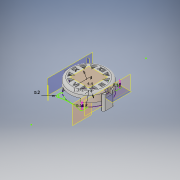
# Autodesk Inventor part: watchBodyOneTopV1.1
Saved by Autodesk Inventor 2019 (Build 230136000, 136)
## iProperties
Created: 2019-10-08
Part Number: watchBodyOneTopV1.1
Material: Generic
Document SubType Name: Modeling
Designer: Derek
Density: 1 g/cm^3
Appearance: Default
Author: Derek
Autodesk Inventor part; units mm, degrees
ref_plane "YZ Plane" through (0, 0, 0) normal (1, 0, 0) x (0, 1, 0)
ref_plane "XZ Plane" through (0, 0, 0) normal (0, 1, 0) x (-1, 0, 0)
ref_plane "XY Plane" through (0, 0, 0) normal (0, 0, 1) x (1, 0, 0)
sketch "Sketch1" plane through (0, 0, 0) normal (0, 1, 0) x (-1, 0, 0)
  circle A0 centre (0, 0) radius 22
  arc A1 (-13.7238, -17.1947) -> (13.7238, -17.1947) centre (0, 0) ccw
  dimension "d0" = 44
  dimension "d11" = 13.7238
  constraints: 4 point on circle, 2 centre point, 1 coincident, 1 concentric
  measures "d0" diameter of A0
  measures "d11" horizontal distance of point (0, 0) A0.start
ref_plane "Work Plane10" through (0, 7, 0) normal (0, 1, 0) x (1, 0, 0)
sketch "Sketch5" plane through (0, 7, 0) normal (0, 1, 0) x (1, 0, 0)
  circle A0 centre (0, 0) radius 20
  dimension "d8" = 40
  constraints: 1 centre point, 1 coincident
  measures "d8" diameter of A0
ref_plane "Work Plane9" through (0, 0, 0) normal (0, -1, 0) x (1, 0, 0)
sketch "Sketch8" plane through (0, 0, 0) normal (0, -1, 0) x (1, 0, 0)
  arc A0 (-11.5874, -18.7011) -> (11.5874, -18.7011) centre (0, 0) ccw
  line L0 (-15.0453, -16.0511) -> (-15.0453, -22.0257)
  line L1 (15.0453, -16.0511) -> (15.0453, -22.0257)
  arc A1 (-15.0453, -16.0511) -> (15.0453, -16.0511) centre (0, 0) ccw
  arc A2 (-15.0453, -22.0257) -> (-13.0453, -24.0257) centre (-13.0453, -22.0257) ccw
  arc A3 (13.0453, -24.0257) -> (15.0453, -22.0257) centre (13.0453, -22.0257) ccw
  line L2 (-15.0451, -16.0514) -> (-15.0451, -22.026)
  arc A4 (-15.0451, -22.026) -> (-13.0451, -24.026) centre (-13.0451, -22.026) ccw
  arc A5 (13.0456, -24.026) -> (15.0456, -22.026) centre (13.0456, -22.026) ccw
  line L3 (15.0456, -16.0514) -> (15.0456, -22.026)
  arc A6 (-15.0451, -16.0514) -> (15.0456, -16.0514) centre (0.0003, -0.0002) ccw
  arc A7 (13.0456, -24.026) -> (-13.0451, -24.026) centre (0.0003, -66.8475) ccw
  point P0 (0, 0)
  point P1 (0, 0)
  constraints: 16 point on circle, 8 centre point, 8 end point
ref_plane "Work Plane8" through (0, 0, 0) normal (0, -1, 0) x (1, 0, 0)
sketch "Sketch11" plane through (0, 0, 0) normal (0, -1, 0) x (1, 0, 0)
  arc A0 (11.5874, 18.7011) -> (-11.5874, 18.7011) centre (0, 0) ccw
  line L0 (-15.0453, 16.0511) -> (-15.0453, 22.0257)
  line L1 (15.0453, 16.0511) -> (15.0453, 22.0257)
  arc A1 (15.0453, 16.0511) -> (-15.0453, 16.0511) centre (0, 0) ccw
  arc A2 (-13.0453, 24.0257) -> (-15.0453, 22.0257) centre (-13.0453, 22.0257) ccw
  arc A3 (15.0453, 22.0257) -> (13.0453, 24.0257) centre (13.0453, 22.0257) ccw
  line L2 (-15.0451, 16.0514) -> (-15.0451, 22.026)
  arc A4 (-13.0451, 24.026) -> (-15.0451, 22.026) centre (-13.0451, 22.026) ccw
  arc A5 (15.0456, 22.026) -> (13.0456, 24.026) centre (13.0456, 22.026) ccw
  line L3 (15.0456, 16.0514) -> (15.0456, 22.026)
  arc A6 (15.0456, 16.0514) -> (-15.0451, 16.0514) centre (0.0003, 0.0002) ccw
  arc A7 (-13.0451, 24.026) -> (13.0456, 24.026) centre (0.0003, 66.8475) ccw
  point P0 (0, 0)
  dimension "d27" = 2
  dimension "d28" = 2
  constraints: 16 point on circle, 8 centre point, 8 end point, 4 tangent, 4 vertical, 2 equal radius
  measures "d27" radius of A2
  measures "d28" radius of A4
ref_plane "Work Plane5" through (14.0456, 0, 22.026) normal (1, 0, 0) x (0, 0, -1)
sketch "Sketch14" plane through (14.0456, 0, 22.026) normal (1, 0, 0) x (0, 0, -1)
  line L0 (0, 0) -> (0, 7) projected
  circle A0 centre (0, 3.5) radius 0.9
  point P0 (22.026, 0)
  dimension "d38" = 1.8
  constraints: 1 centre point, 1 midpoint
  measures "d38" diameter of A0
ref_plane "Work Plane6" through (14.0456, 0, 22.026) normal (1, 0, 0) x (0, 0, -1)
sketch "Sketch15" plane through (14.0456, 0, 22.026) normal (1, 0, 0) x (0, 0, -1)
  line L0 (44.1089, 7) -> (44.1089, 0) projected
  circle A0 centre (44.1089, 3.5) radius 0.9
  point P0 (22.026, 0)
  dimension "d41" = 1.8
  constraints: 1 centre point, 1 midpoint
  measures "d41" diameter of A0
ref_plane "Work Plane7" through (0, 7, 0) normal (0, 1, 0) x (1, 0, 0)
sketch "Sketch16" plane through (0, 7, 0) normal (0, 1, 0) x (1, 0, 0)
  circle A0 centre (0, 0) radius 22
  circle A1 centre (0, -0.3745) radius 18.85
  dimension "d44" = 37.7
  constraints: 2 centre point, 1 coincident
  measures "d44" diameter of A1
extrude "Extrusion13" add sketch "Sketch16" along normal blind 7.5
ref_plane "Work Plane3" through (22, 0, 0) normal (1, 0, 0) x (0, 1, 0)
sketch "Sketch17" plane through (22, 0, 0) normal (1, 0, 0) x (0, 1, 0)
  line L0 (7, -18.2255) -> (7, 18.9745) projected
  line L1 (11.1125, 6.35) -> (7, 6.35)
  line L2 (7, 6.35) -> (7, -6.5465)
  line L3 (7, -6.5465) -> (11.1125, -6.5465)
  line L4 (11.1125, -6.5465) -> (11.1125, 6.35)
  constraints: 8 end point, 2 parallel, 1 horizontal, 1 perpendicular, 1 point on line
extrude "Extrusion14" add sketch "Sketch17" along normal mid plane 3
ref_plane "Work Plane12" through (21.0034, 7, -6.5465) normal (0, -1, 0) x (1, 0, 0)
sketch "Sketch18" plane through (21.0034, 7, -6.5465) normal (0, -1, 0) x (1, 0, 0)
  arc A0 (-35.8073, -9.7276) -> (-35.8073, 22.8206) centre (-21.0034, 6.5465) ccw projected
  line L0 (0, 0) -> (2.4966, 0) projected
  line L1 (0, 0) -> (2.4966, 0)
  line L2 (2.4966, 12.8965) -> (0.0602, 12.8965) projected
  line L3 (2.4966, 0) -> (2.4966, 12.8965)
  line L4 (2.4966, 12.8965) -> (0.0602, 12.8965)
  arc A1 (0, 0) -> (0.0602, 12.8965) centre (-21.0034, 6.5465) ccw
  constraints: 6 end point, 3 point on circle, 2 collinear, 1 centre point, 1 perpendicular
extrude "Extrusion15" add sketch "Sketch18" along normal blind 12.8
ref_plane "Work Plane4" through (-22, 0, 0) normal (-1, 0, 0) x (0, -1, 0)
sketch "Sketch19" plane through (-22, 0, 0) normal (-1, 0, 0) x (0, -1, 0)
  line L0 (-11.1125, -6.5465) -> (-11.1125, 6.35) projected
  line L1 (-7, -20) -> (-7, 20) projected
  line L2 (-11.1125, -6.5465) -> (-7, -6.5465)
  line L3 (-7, -6.5465) -> (-7, 6.35)
  line L4 (-7, 6.35) -> (-11.1125, 6.35)
  line L5 (-11.1125, 6.35) -> (-11.1125, -6.5465)
  point P0 (0, 0)
  constraints: 8 end point, 2 parallel, 1 horizontal, 1 perpendicular, 1 point on line
extrude "Extrusion16" add sketch "Sketch19" along normal mid plane 3
sketch "Sketch20" plane through (-23.5, 7, -6.5465) normal (0, -1, 0) x (1, 0, 0)
  line L0 (0, 0) -> (2.4966, 0) projected
  line L1 (2.4966, 0) -> (0, 0)
  line L2 (0, 12.8965) -> (0, 0) projected
  line L3 (0, 0) -> (0, 12.8965)
  arc A0 (2.4363, 12.8965) -> (2.4966, 0) centre (23.5, 6.5465) ccw projected
  line L4 (0, 12.8965) -> (2.4363, 12.8965)
  point P0 (3, 0)
  constraints: 6 end point, 2 collinear, 1 perpendicular
extrude "Extrusion17" add sketch "Sketch20" along normal blind 12.8
ref_plane "Work Plane11" through (0, 14.5, 0) normal (0, 1, 0) x (1, 0, 0)
sketch "Sketch23" plane through (0, 14.5, 0) normal (0, 1, 0) x (1, 0, 0)
  circle A0 centre (0, 0) radius 20
  constraints: 1 centre point, 1 coincident
extrude "Extrusion20" add sketch "Sketch23" against normal blind 2
fillet "Fillet1" radius 3 1 edges at (-22, 14.5, 0)
ref_plane "Work Plane13" through (-21.0034, 11.1125, -21.5465) normal (0, 0, -1) x (-1, 0, 0)
sketch "Sketch36" plane through (23.5, 0, 0) normal (1, 0, 0) x (0, 0, -1)
  line L0 (3.8069, 13.5118) -> (-2.6931, 13.5118)
  line L1 (-2.6931, 13.5118) -> (-2.6931, 7.0118)
  line L2 (-2.6931, 7.0118) -> (3.8069, 7.0118)
  line L3 (3.8069, 7.0118) -> (3.8069, 13.5118)
  point P0 (0, 0)
  dimension "d96" = 6.5
  dimension "d97" = 6.5
  constraints: 8 end point, 2 parallel, 1 horizontal, 1 perpendicular
  measures "d96" distance of L2.end L1.end
  measures "d97" distance of L1.end L0.end
extrude "Extrusion26" cut sketch "Sketch36" against normal blind 5
sketch "Sketch37" plane through (18.5, 0, 0) normal (1, 0, 0) x (0, 0, -1)
  line L0 (3.8069, 13.5118) -> (3.8069, 7.0118) projected
  line L1 (3.8069, 13.5118) -> (-2.6931, 13.5118) projected
  line L2 (3.8069, 7.0118) -> (-2.6931, 7.0118)
  line L3 (-2.6931, 7.0118) -> (-2.6931, 13.5118)
  line L4 (-2.6931, 13.5118) -> (3.8069, 13.5118)
  line L5 (3.8069, 13.5118) -> (3.8069, 7.0118)
  point P0 (0, 0)
  constraints: 8 end point, 2 parallel, 1 horizontal, 1 perpendicular
extrude "Extrusion27" cut sketch "Sketch37" against normal blind 5
fillet "Fillet2" radius 2 1 edges at (-23.5, 2.6562, -6.5465)
fillet "Fillet3" radius 2 1 edges at (-23.5, 2.6562, 6.35)
fillet "Fillet4" radius 2 2 edges at (23.5, 2.6562, 6.35) (23.5, 2.6562, -6.5465)
ref_plane "Work Plane14" through (-21.0637, -5.8, 26.35) normal (0, 0, 1) x (1, 0, 0)
sketch "Sketch39" plane through (0, 7, 0) normal (0, -1, 0) x (1, 0, 0)
  circle A0 centre (0, 0) radius 20
  circle A1 centre (0, 0) radius 19 projected
  circle A2 centre (0, 0) radius 22
  constraints: 2 centre point, 2 coincident
extrude "Extrusion30" add sketch "Sketch39" along normal blind 3 contours A2
sketch "Sketch40" plane through (-21.0637, -5.8, 26.35) normal (0, 0, 1) x (1, 0, 0)
  line L0 (0.0602, 9.8) -> (42.0671, 9.8) projected
  line L1 (31.2191, 9.8) -> (10.2191, 9.8)
  line L2 (10.2191, 9.8) -> (10.2191, 13.8)
  line L3 (10.2191, 13.8) -> (31.2191, 13.8)
  line L4 (31.2191, 13.8) -> (31.2191, 9.8)
  point P0 (21.0637, 5.8)
  dimension "d115" = 21
  dimension "d116" = 4
  constraints: 8 end point, 2 parallel, 1 horizontal, 1 perpendicular, 1 point on line
  measures "d115" distance of L2.end L3.end
  measures "d116" distance of L1.end L2.end
extrude "Extrusion31" cut sketch "Sketch40" against normal blind 12
sketch "Sketch24" plane through (0, 14.5, 0) normal (0, 1, 0) x (1, 0, 0)
  line L0 (10.9767, 13.2796) -> (5.8224, 10.3341)
  line L1 (5.8224, 10.3341) -> (5.8486, 16.2706)
  line L2 (5.8486, 16.2706) -> (10.9767, 13.2796)
  line L3 (16.5131, 5.8755) -> (10.4909, 5.9199)
  line L4 (10.4909, 5.9199) -> (13.5405, 11.113)
  line L5 (13.5405, 11.113) -> (16.5131, 5.8755)
  line L6 (16.5966, -6.2702) -> (13.432, -11.5016)
  line L7 (13.432, -11.5016) -> (10.4838, -6.1453)
  line L8 (10.4838, -6.1453) -> (16.5966, -6.2702)
  line L9 (11.4269, -13.3864) -> (6.4692, -16.6726)
  line L10 (6.4692, -16.6726) -> (6.1021, -10.736)
  line L11 (6.1021, -10.736) -> (11.4269, -13.3864)
  line L12 (-6.0129, -10.6804) -> (-5.9694, -16.6431)
  line L13 (-5.9694, -16.6431) -> (-11.155, -13.6995)
  line L14 (-11.155, -13.6995) -> (-6.0129, -10.6804)
  line L15 (-10.2253, -6.1862) -> (-13.3868, -11.6656)
  line L16 (-13.3868, -11.6656) -> (-16.5514, -6.188)
  line L17 (-16.5514, -6.188) -> (-10.2253, -6.1862)
  line L18 (-10.6525, 5.6862) -> (-16.9579, 5.7959)
  line L19 (-16.9579, 5.7959) -> (-13.7102, 11.2018)
  line L20 (-13.7102, 11.2018) -> (-10.6525, 5.6862)
  line L21 (-6.1885, 9.9631) -> (-11.4992, 13.2741)
  line L22 (-11.4992, 13.2741) -> (-5.9764, 16.2178)
  line L23 (-5.9764, 16.2178) -> (-6.1885, 9.9631)
  line L24 (-3.7539, 17.3089) -> (3.62, 17.3089) construction
  line L25 (3.62, 17.3089) -> (3.62, 12.7336) construction
  line L26 (3.62, 12.7336) -> (-3.7539, 12.7336) construction
  line L27 (-3.7539, 12.7336) -> (-3.7539, 17.3089) construction
  line L28 (5.558, 19.0366) -> (5.558, 14.4613) construction
  line L29 (12.8351, 2.0932) -> (17.8398, 2.0932) construction
  line L30 (17.8398, 2.0932) -> (17.8398, -2.2068) construction
  line L31 (17.8398, -2.2068) -> (12.8351, -2.2068) construction
  line L32 (12.8351, -2.2068) -> (12.8351, 2.0932) construction
  line L33 (-2.7032, -13.1458) -> (2.3586, -13.1458) construction
  line L34 (2.3586, -13.1458) -> (2.3586, -17.8139) construction
  line L35 (2.3586, -17.8139) -> (-2.7032, -17.8139) construction
  line L36 (-2.7032, -17.8139) -> (-2.7032, -13.1458) construction
  line L37 (-18.4501, 2.0895) -> (-13.3883, 2.0895) construction
  line L38 (-13.3883, 2.0895) -> (-13.3883, -2.5786) construction
  line L39 (-13.3883, -2.5786) -> (-18.4501, -2.5786) construction
  line L40 (-18.4501, -2.5786) -> (-18.4501, 2.0895) construction
  line L41 (-18.0404, -2.2105) -> (-18.0404, 2.0895)
  line L42 (-18.0404, 2.0895) -> (-17.1719, 2.0895)
  line L43 (-17.1719, 2.0895) -> (-17.1719, -2.2105)
  line L44 (-17.1719, -2.2105) -> (-18.0404, -2.2105)
  line L45 (-16.7786, -2.2105) -> (-15.294, 0.0279)
  line L46 (-15.294, 0.0279) -> (-16.641, 2.0895)
  line L47 (-16.641, 2.0895) -> (-15.6283, 2.0895)
  line L48 (-15.6283, 2.0895) -> (-14.7761, 0.8047)
  line L49 (-14.7761, 0.8047) -> (-13.924, 2.0895)
  line L50 (-13.924, 2.0895) -> (-12.9113, 2.0895)
  line L51 (-12.9113, 2.0895) -> (-14.2648, 0.0312)
  line L52 (-14.2648, 0.0312) -> (-12.7802, -2.2105)
  line L53 (-12.7802, -2.2105) -> (-13.8289, -2.2105)
  line L54 (-13.8289, -2.2105) -> (-14.7827, -0.7554)
  line L55 (-14.7827, -0.7554) -> (-15.7364, -2.2105)
  line L56 (-15.7364, -2.2105) -> (-16.7786, -2.2105)
  line L57 (-3.736, 13.0089) -> (-2.2514, 15.2474)
  line L58 (-2.2514, 15.2474) -> (-3.5984, 17.3089)
  line L59 (-3.5984, 17.3089) -> (-2.5857, 17.3089)
  line L60 (-2.5857, 17.3089) -> (-1.7335, 16.0242)
  line L61 (-1.7335, 16.0242) -> (-0.8814, 17.3089)
  line L62 (-0.8814, 17.3089) -> (0.1313, 17.3089)
  line L63 (0.1313, 17.3089) -> (-1.2222, 15.2507)
  line L64 (-1.2222, 15.2507) -> (0.2624, 13.0089)
  line L65 (0.2624, 13.0089) -> (-0.7863, 13.0089)
  line L66 (-0.7863, 13.0089) -> (-1.7401, 14.4641)
  line L67 (-1.7401, 14.4641) -> (-2.6938, 13.0089)
  line L68 (-2.6938, 13.0089) -> (-3.736, 13.0089)
  line L69 (0.6787, 13.0089) -> (0.6787, 17.3089)
  line L70 (0.6787, 17.3089) -> (1.5472, 17.3089)
  line L71 (1.5472, 17.3089) -> (1.5472, 13.0089)
  line L72 (1.5472, 13.0089) -> (0.6787, 13.0089)
  line L73 (2.3469, 13.0089) -> (2.3469, 17.3089)
  line L74 (2.3469, 17.3089) -> (3.2154, 17.3089)
  line L75 (3.2154, 17.3089) -> (3.2154, 13.0089)
  line L76 (3.2154, 13.0089) -> (2.3469, 13.0089)
  line L77 (13.2448, -2.2068) -> (13.2448, 2.0932)
  line L78 (13.2448, 2.0932) -> (14.1133, 2.0932)
  line L79 (14.1133, 2.0932) -> (14.1133, -2.2068)
  line L80 (14.1133, -2.2068) -> (13.2448, -2.2068)
  line L81 (14.913, -2.2068) -> (14.913, 2.0932)
  line L82 (14.913, 2.0932) -> (15.7816, 2.0932)
  line L83 (15.7816, 2.0932) -> (15.7816, -2.2068)
  line L84 (15.7816, -2.2068) -> (14.913, -2.2068)
  line L85 (16.5813, -2.2068) -> (16.5813, 2.0932)
  line L86 (16.5813, 2.0932) -> (17.4498, 2.0932)
  line L87 (17.4498, 2.0932) -> (17.4498, -2.2068)
  line L88 (17.4498, -2.2068) -> (16.5813, -2.2068)
  line L89 (-1.1661, -17.4458) -> (-2.7032, -13.1458)
  line L90 (-2.7032, -13.1458) -> (-1.7626, -13.1458)
  line L91 (-1.7626, -13.1458) -> (-0.6712, -16.3282)
  line L92 (-0.6712, -16.3282) -> (0.3808, -13.1458)
  line L93 (0.3808, -13.1458) -> (1.3018, -13.1458)
  line L94 (1.3018, -13.1458) -> (-0.2353, -17.4458)
  line L95 (-0.2353, -17.4458) -> (-1.1661, -17.4458)
  line L96 (1.7148, -17.4458) -> (1.7148, -13.1458)
  line L97 (1.7148, -13.1458) -> (2.5833, -13.1458)
  line L98 (2.5833, -13.1458) -> (2.5833, -17.4458)
  line L99 (2.5833, -17.4458) -> (1.7148, -17.4458)
  point P0 (0, 0)
  point P1 (7.5492, 13.2948)
  point P2 (13.5148, 7.6361)
  point P3 (13.5041, -7.9724)
  point P4 (7.9994, -13.5983)
  point P5 (-7.7124, -13.6743)
  point P6 (-13.3879, -8.0132)
  point P7 (-13.7736, 7.5613)
  point P8 (-7.888, 13.1517)
  constraints: 48 end point, 64 other
extrude "Extrusion32" cut sketch "Sketch24" against normal blind 3
body "Solid1"
